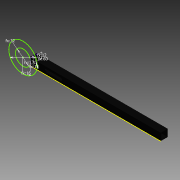
# Autodesk Inventor part: KétvégenMartSzelvény
Saved by Autodesk Inventor 2015 SP1 (Build 190203100, 203)
## iProperties
Created: 2014-08-08
Part Number: KétvégenMartSzelvény
Material: Acetal Resin, Black
Document SubType Name: Modeling
Designer: laca
Density: 1.425 g/cm^3
Appearance: Smooth - Black
Mass: 61.9349 g
Surface Area: 586.029 cm^2
Volume: 43.4631 cm^3
FalVastagsag: 1.500 mm
BelsoAtmero: 12.000 mm
d2: 12.000 mm
d3: 275.000 mm
d4: 0.00 deg
d8: 32.000 mm
d9: 16.000 mm
d12: 10.000 mm
d13: 0.00 deg
d15: 0.00 deg
ZártSzelvényFalVastagság: 1.500 mm
ZártSzelvényBelsőÁtmérő: 12.000 mm
CsapágyHázKülsőÁtmérő: 32.000 mm
ZártSzelvényKülsőÁtmérő: 15.000 mm
CsapágyBelsőÁtmérő: 12.000 mm
CsapágyKülsőÁtmérő: 28.000 mm
CsapágyHázBelsőÁtmérő: 26.000 mm
CTipHoszza: 400.000 mm
ATipHoszza: 400.000 mm
BTipHoszza: 70.000 mm
CsapágyHázHoszza: 45.000 mm
CsapágySzélesége: 8.000 mm
Author: laca
Autodesk Inventor part; units mm, degrees
ref_plane "YZ Plane" through (0, 0, 0) normal (1, 0, 0) x (0, 1, 0)
ref_plane "XZ Plane" through (0, 0, 0) normal (0, 1, 0) x (-1, 0, 0)
ref_plane "XY Plane" through (0, 0, 0) normal (0, 0, 1) x (1, 0, 0)
sketch "Sketch1" plane through (0, 0, 0) normal (1, 0, 0) x (0, 1, 0)
  line L0 (0, 0) -> (12, 0)
  line L1 (12, 0) -> (12, 12)
  line L2 (12, 12) -> (0, 12)
  line L3 (0, 12) -> (0, 0)
  line L4 (-1.5, 13.5) -> (13.5, 13.5)
  line L5 (13.5, 13.5) -> (13.5, -1.5)
  line L6 (13.5, -1.5) -> (-1.5, -1.5)
  line L7 (-1.5, -1.5) -> (-1.5, 13.5)
  dimension "FalVastagsag" = 1.5
  dimension "BelsoAtmero" = 12
  dimension "d2" = 12
  constraints: 16 end point, 4 parallel, 2 perpendicular, 1 horizontal, 3 other
  measures "FalVastagsag" distance between parallel lines of L4 L2
  measures "BelsoAtmero" distance of L2.end L0.start
  measures "d2" distance of L0.start L0.end
extrude "Extrusion1" add sketch "Sketch1" along normal blind 275
sketch "Sketch2" plane through (0, -1.5, 13.5) normal (0, 0, 1) x (1, 0, 0)
  line L0 (0, 0) -> (0, 15) projected
  line L1 (0, 0) -> (275, 0) projected
  circle A0 centre (-16, 7.5) radius 16
  circle A1 centre (-16, 7.5) radius 30
  circle A2 centre (14, 7.5) radius 2
  point P0 (0, 1.5)
  dimension "d22" = 60
  dimension "d8" = 32
  dimension "d9" = 16
  dimension "d23" = 4
  constraints: 2 centre point, 1 coincident, 1 horizontal alignment, 2 other
  measures "d8" diameter of A0
  measures "d9" distance from line of L0 A0.centre
  measures "d23" diameter of A2
sketch "Sketch4" plane through (0, 0, 0) normal (-1, 0, 0) x (0, 0, 1)
  line L0 (0, 0) -> (12, 0)
  line L1 (12, 0) -> (12, 12)
  line L2 (12, 12) -> (0, 12)
  line L3 (0, 12) -> (0, 0)
  line L4 (-1.5, -1.5) -> (13.5, -1.5)
  line L5 (13.5, -1.5) -> (13.5, 13.5)
  line L6 (13.5, 13.5) -> (-1.5, 13.5)
  line L7 (-1.5, 13.5) -> (-1.5, -1.5)
  constraints: 16 end point, 4 parallel, 2 horizontal, 2 perpendicular
extrude "Extrusion2" add sketch "Sketch4" along normal blind 10
extrude "Extrusion3" cut sketch "Sketch2" against normal through all contours A0
sketch "Sketch5" plane through (-16, 6, 13.5) normal (0, 0, 1) x (1, 0, 0)
  arc A0 (50, 2.9901) -> (50, -3.0099) centre (50, -0.0099) ccw
  arc A1 (80, -3.0099) -> (80, 2.9901) centre (80, -0.0099) ccw
  line L0 (50, 2.9901) -> (80, 2.9901)
  line L1 (80, -3.0099) -> (50, -3.0099)
  arc A2 (14.1333, -7.5) -> (14.1333, 7.5) centre (0, 0) ccw projected
  point P0 (16, -6)
  dimension "d16" = 6
  dimension "d17" = 6
  dimension "d18" = 30
  dimension "d19" = 50
  constraints: 4 end point, 4 point on circle, 3 tangent, 2 centre point
  measures "d16" diameter of A0
  measures "d17" diameter of A1
  measures "d18" distance of A1.centre A0.centre
  measures "d19" distance of A2.centre A0.centre
extrude "Extrusion4" cut sketch "Sketch5" against normal through all
extrude "Extrusion5" cut sketch "Sketch2" against normal through all contours A1 A2 | A1 A2 picked at (13.3724, 7.0462) picked at (14.5954, 6.9828)
mirror "Mirror2" [suppressed]
equation "\"FalVastagsag\" = ZártSzelvényFalVastagság"
equation "\"BelsoAtmero\" = ZártSzelvényBelsőÁtmérő"
equation "\"d2\" = ZártSzelvényBelsőÁtmérő"
equation "\"d22\" = 2 * PorvedoRogzitesJatekSugara"
equation "\"d8\" = CsapágyHázKülsőÁtmérő"
equation "\"d9\" = 0.5 * CsapágyHázKülsőÁtmérő"
equation "\"ZártSzelvényFalVastagság\" = 1.5"
equation "\"ZártSzelvényBelsőÁtmérő\" = 12"
equation "\"CsapágyHázKülsőÁtmérő\" = 32"
equation "\"ZártSzelvényKülsőÁtmérő\" = 15"
equation "\"CsapágyBelsőÁtmérő\" = 12"
equation "\"CsapágyKülsőÁtmérő\" = 28"
equation "\"CsapágyHázBelsőÁtmérő\" = 26"
equation "\"CTipHoszza\" = 400"
equation "\"ATipHoszza\" = 400"
equation "\"BTipHoszza\" = 70"
equation "\"CsapágyHázHoszza\" = 45"
equation "\"CsapágySzélesége\" = 8"
equation "\"PorvedoRogzitesJatekSugara\" = 30"
body "Solid1"
